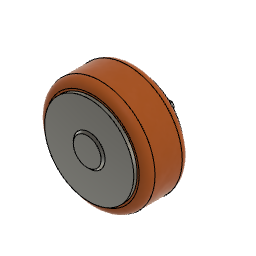
BEAST - Cart (Autodesk Fusion 360 archive; units mm, degrees)
design "ZLLG65ASM500"
Autodesk Fusion 360 part; units mm, degrees
cylinder "CylinderPrimitive1" add diameter 135 height 75.5 placed x (1, 0, 0) y (0, 0, -1) z (0, 1, 0) at (0, 0, 0) makes body 1
cylinder "CylinderPrimitive2" add diameter 48 height -3 placed x (1, 0, 0) y (0, 0, -1) z (0, 1, 0) at (0, 0, 0) bodies 1
cylinder "CylinderPrimitive3" add diameter 48 height 3 placed x (1, 0, 0) y (0, 0, -1) z (0, 1, 0) at (0, 75.5, 0) bodies 1
chamfer "Chamfer1" distance 3 angle 45 2 edges at (-22.3759, 78.5, 8.6788) (-8.6788, -3, 22.3759) on bodies 1
cylinder "CylinderPrimitive4" add diameter 165 height 65.2 placed x (1, 0, 0) y (0, 0, -1) z (0, 1, 0) at (0, 0, 0) separate body makes body 2
cylinder "CylinderPrimitive5" cut diameter 135 height -130 placed x (1, 0, 0) y (0, 0, 1) z (0, -1, 0) at (0, 0, 0) bodies 2
fillet "Fillet1" radius 12 2 edges at (-76.917, 0, -29.8333) (-76.917, 65.2, 29.8333) on bodies 2
move_body "Align1" bodies 2 to x (1, 0, 0) y (0, 1, 0) z (0, 0, 1) at (0, 5.15, 0)
cylinder "CylinderPrimitive6" add diameter 16 height 42 placed x (1, 0, 0) y (0, 0, -1) z (0, 1, 0) at (0, 78.5, 0) bodies 1
thread "Thread1" "ISO Metric profile 16.0 M16x2 6g" major diameter 15.822 minor diameter 13.534 pitch 2 angle 60 resizes the face on face at (7.9602, 92.5, 0.7965) from (0, 81.5, 0) to (0, 120.5, 0) on bodies 1
sketch "Sketch9" plane through (0, 120.5, 0) normal (0, 1, 0) x (-1, 0, 0)
  circle A0 centre (0, 0) radius 7.911
  line L0 (-10, 6) -> (10, 6)
  line L1 (10, 6) -> (10, 10)
  line L2 (10, 10) -> (-10, 10)
  line L3 (-10, 10) -> (-10, 6)
  line L4 (-10, -6) -> (10, -6)
  line L5 (10, -6) -> (10, -10)
  line L6 (10, -10) -> (-10, -10)
  line L7 (-10, -10) -> (-10, -6)
  constraint horizontal L0
  constraint vertical L1
  constraint horizontal L2
  constraint vertical L3
  constraint horizontal L4
  constraint vertical L5
  constraint horizontal L6
  constraint vertical L7
extrude "Extrude1" cut sketch "Sketch9" against normal blind 39 contours A0 L0 | A0 L4 bodies 1
named bodies: "Hub", "Tyre"
